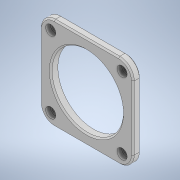
# Autodesk Inventor part: StageInsert_FoilHolder_Part1
Saved by Autodesk Inventor 2026 (Build 300175050, 175E)
## iProperties
Created: 2024-11-14
Part Number: StageInsert_FoilHolder_Part1
Material: Generisch
Document SubType Name: Modeling
Designer: neuhau0004
Density: 1 g/cm^3
Appearance: Vorgabe
Author: neuhau0004
Autodesk Inventor part; units mm, degrees
ref_plane "YZ Plane" through (0, 0, 0) normal (1, 0, 0) x (0, 1, 0)
ref_plane "XZ Plane" through (0, 0, 0) normal (0, 1, 0) x (-1, 0, 0)
ref_plane "XY Plane" through (0, 0, 0) normal (0, 0, 1) x (1, 0, 0)
sketch "Skizze1" plane through (0, 0, 0) normal (0, 0, 1) x (1, 0, 0)
  circle A0 centre (0, 0) radius 25
  line L0 (-32.5, 32.5) -> (32.5, 32.5)
  line L1 (32.5, 22.5) -> (32.5, -22.5)
  line L2 (22.5, -32.5) -> (-22.5, -32.5)
  line L3 (-32.5, -22.5) -> (-32.5, 22.5)
  line L4 (-32.5, 32.5) -> (32.5, -32.5) construction
  line L5 (32.5, 32.5) -> (-32.5, -32.5) construction
  circle A1 centre (-25, 25) radius 2.1
  circle A2 centre (25, 25) radius 2.1
  circle A3 centre (-25, -25) radius 2.1
  circle A4 centre (25, -25) radius 2.1
  line L6 (-22.5, 32.5) -> (22.5, 32.5)
  line L7 (32.5, -32.5) -> (-32.5, -32.5)
  line L8 (-32.5, -32.5) -> (-32.5, 32.5)
  line L9 (32.5, 32.5) -> (32.5, -32.5)
  arc A5 (-22.5, 32.5) -> (-32.5, 22.5) centre (-22.5, 22.5) ccw
  arc A6 (-32.5, -22.5) -> (-22.5, -32.5) centre (-22.5, -22.5) ccw
  arc A7 (22.5, -32.5) -> (32.5, -22.5) centre (22.5, -22.5) ccw
  arc A8 (32.5, 22.5) -> (22.5, 32.5) centre (22.5, 22.5) ccw
  dimension "d0" = 50
  dimension "d1" = 65
  dimension "d2" = 65
  dimension "d5" = 25
  dimension "d6" = 25
  dimension "d7" = 4.2
  dimension "d10" = 50
  dimension "d13" = 50
  dimension "d16" = 10
  constraints: 20 end point, 9 centre point, 9 point on line, 8 point on circle, 8 tangent, 3 equal radius, 3 perpendicular, 2 coincident, 2 horizontal, 2 midpoint, 2 parallel, 1 collinear, 1 vertical, 6 other
  measures "d0" diameter of A0
  measures "d1" distance of L4.end L5.end
  measures "d2" distance of L0.end L4.end
  measures "d5" horizontal distance of point (0, 0) point (-25, 25)
  measures "d6" horizontal distance of point (0, 0) point (-25, 25)
  measures "d7" diameter of A1
  measures "d10" distance of A1.centre A2.centre
  measures "d13" distance of A1.centre A3.centre
  measures "d16" radius of A5
extrude "Extrusion1" add sketch "Skizze1" along normal blind 5 contours L0 A8 L1 A7 L2 A6 L3 A5
sketch "Skizze2" plane through (0, 0, 5) normal (0, 0, 1) x (1, 0, 0)
  circle A0 centre (-25, 25) radius 2.1 projected
  circle A1 centre (-25, 25) radius 3.525
  circle A2 centre (25, 25) radius 2.1 projected
  circle A3 centre (25, 25) radius 3.525
  circle A4 centre (-25, -25) radius 2.1 projected
  circle A5 centre (-25, -25) radius 3.525
  circle A6 centre (25, -25) radius 2.1 projected
  circle A7 centre (25, -25) radius 3.525
  point P0 (0, 0)
  dimension "d17" = 7.05
  dimension "d18" = 7.05
  dimension "d19" = 7.05
  dimension "d20" = 7.05
  constraints: 4 centre point, 4 coincident
  measures "d17" diameter of A1
  measures "d18" diameter of A3
  measures "d19" diameter of A5
  measures "d20" diameter of A7
extrude "Extrusion2" cut sketch "Skizze2" against normal blind 3.2
chamfer "Fase1" distance 1 angle 45 9 edges at (-25, 0, 5) (0, -32.5, 5) (29.5711, -29.5711, 5) (32.5, 0, 5) (29.5711, 29.5711, 5) (0, 32.5, 5) (-29.5711, 29.5711, 5) (-32.5, 0, 5) (-29.5711, -29.5711, 5)
chamfer "Fase2" distance 0.5 angle 45 8 edges at (0, 32.5, 0) (-29.5711, 29.5711, 0) (-32.5, 0, 0) (-29.5711, -29.5711, 0) (0, -32.5, 0) (29.5711, -29.5711, 0) (32.5, 0, 0) (29.5711, 29.5711, 0)
